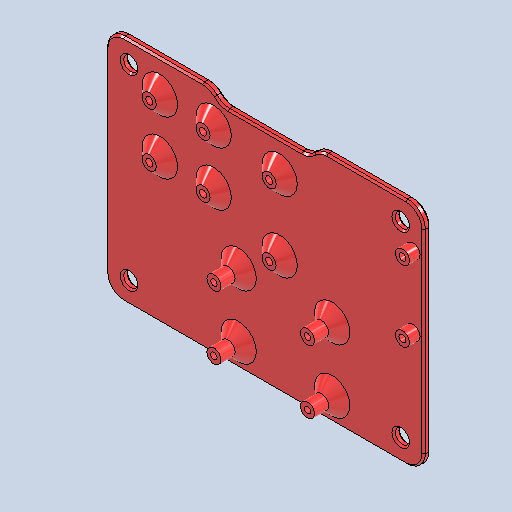
# Autodesk Inventor part: temp-logger-shelf-v2
Saved by Autodesk Inventor 2026 (Build 300175050, 175E)
## iProperties
Created: 2025-07-16
Part Number: temp-logger-shelf-v2
Material: ABS Plastic
Document SubType Name: Modeling
Designer: kuzmin
Density: 1.06 g/cm^3
Appearance: Light Red
Author: kuzmin
Autodesk Inventor part; units mm, degrees
ref_plane "YZ Plane" through (0, 0, 0) normal (1, 0, 0) x (0, 1, 0)
ref_plane "XZ Plane" through (0, 0, 0) normal (0, 1, 0) x (-1, 0, 0)
ref_plane "XY Plane" through (0, 0, 0) normal (0, 0, 1) x (1, 0, 0)
sketch "Sketch1" plane through (0, 0, 0) normal (0, 0, 1) x (1, 0, 0)
  line L0 (-45, 32.5) -> (45, 32.5)
  line L1 (45, 32.5) -> (45, -32.5)
  line L2 (45, -32.5) -> (-45, -32.5)
  line L3 (-45, -32.5) -> (-45, 32.5)
  line L4 (-38.5, 26.5) -> (38.5, 26.5) construction
  line L5 (38.5, 26.5) -> (38.5, -26.5) construction
  line L6 (38.5, -26.5) -> (-38.5, -26.5) construction
  line L7 (-38.5, -26.5) -> (-38.5, 26.5) construction
  circle A0 centre (-38.5, 26.5) radius 2
  circle A1 centre (38.5, 26.5) radius 2
  circle A2 centre (38.5, -26.5) radius 2
  circle A3 centre (-38.5, -26.5) radius 2
  point P0 (0, 0)
  point P1 (45, 0)
  point P2 (0, 32.5)
  point P3 (38.5, 0)
  point P4 (0, 26.5)
  dimension "d0" = 90
  dimension "d1" = 65
  dimension "d2" = 77
  dimension "d3" = 53
  dimension "d14" = 4
  constraints: 16 end point, 8 coincident, 4 centre point, 4 midpoint, 4 parallel, 3 equal radius, 2 horizontal, 2 horizontal alignment, 2 perpendicular, 2 vertical alignment
  measures "d0" distance of L0.start L0.end
  measures "d1" distance of L0.end L1.end
  measures "d2" distance of L4.start L4.end
  measures "d3" distance of L4.end L5.end
  measures "d14" diameter of A0
extrude "Extrusion1" add sketch "Sketch1" along normal blind 2 contours L0 L1 L2 L3 | A0 | A1 | A2 | A3
hole "Hole1" at (38.5, 26.5, 0) at (38.5, -26.5, 0) at (-38.5, -26.5, 0) at (-38.5, 26.5, 0) direction (0, 0, 1) diameter 4 end through all
sketch "Sketch3" plane through (0, 0, 0) normal (0, 0, -1) x (-1, 0, 0)
  line L0 (-42, 21) -> (-4.2, 21) construction
  line L1 (-4.2, 21) -> (-4.2, 1) construction
  line L2 (-4.2, 1) -> (-42, 1) construction
  line L3 (-42, 1) -> (-42, 21) construction
  circle A0 centre (-42, 21) radius 2
  circle A1 centre (-4.2, 21) radius 2
  circle A2 centre (-4.2, 1) radius 2
  circle A3 centre (-42, 1) radius 2
  line L4 (-40, -32.5) -> (40, -32.5) projected
  line L5 (-45, -32.5) -> (-45, 32.5) projected
  point P0 (0, 0)
  point P1 (-4.2, 11)
  point P2 (-45, -27.5)
  point P3 (-45, 27.5)
  dimension "d27" = 20
  dimension "d28" = 37.8
  dimension "d30" = 4
  dimension "d47" = 3
  dimension "d107" = 21
  constraints: 8 coincident, 8 end point, 4 centre point, 3 equal radius, 2 parallel, 1 horizontal, 1 midpoint, 1 perpendicular
  measures "d27" distance of L0.end L1.end
  measures "d28" distance of L0.start L0.end
  measures "d30" diameter of A1
  measures "d47" distance between parallel lines of L5 L3
  measures "d107" distance from line of point (0, 0) L0
extrude "Extrusion4" add sketch "Sketch3" against normal blind 5
hole "Hole2" at (4.2, 21, 0) at (4.2, 1, 0) at (42, 1, 0) at (42, 21, 0) direction (0, 0, 1) diameter 2 end through all
sketch "Sketch8" plane through (0, 0, 2) normal (0, 0, 1) x (1, 0, 0)
  line L0 (45, 32.5) -> (-45, 32.5) projected
  line L1 (-15, 32.5) -> (15, 32.5)
  line L2 (15, 32.5) -> (15, 29.5)
  line L3 (15, 29.5) -> (-15, 29.5)
  line L4 (-15, 29.5) -> (-15, 32.5)
  point P0 (0, 0)
  point P1 (0, 29.5)
  dimension "d108" = 30
  dimension "d109" = 3
  constraints: 8 end point, 2 parallel, 1 horizontal, 1 midpoint, 1 perpendicular, 1 point on line, 1 vertical alignment
  measures "d108" distance of L2.end L3.end
  measures "d109" distance of L3.end L1.start
extrude "Extrusion10" cut sketch "Sketch8" against normal through all
chamfer "Chamfer3" distance 3 angle 45 2 edges at (6.2, 21, 2) (6.2, 1, 2)
fillet "Fillet2" radius 5 8 edges at (-45, 32.5, 1) (-45, -32.5, 1) (45, -32.5, 1) (45, 32.5, 1) (-15, 32.5, 1) (-15, 29.5, 1) (15, 29.5, 1) (15, 32.5, 1)
chamfer "Chamfer5" distance 0.5 angle 45 34 edges at (0, -32.5, 2) (43.5355, -31.0355, 2) (-43.5355, -31.0355, 2) (12.3539, 29.8902, 2) (15.6224, 32.1098, 2) (43.5355, 31.0355, 2) (-43.5355, 31.0355, 2) (-15.6224, 32.1098, 2) (-12.3539, 29.8902, 2) (45, 0, 2) (28.7794, 32.5, 2) (-28.7794, 32.5, 2) (-45, 0, 2) (43.5355, 31.0355, 0) (28.7794, 32.5, 0) (-28.7794, 32.5, 0) (-43.5355, 31.0355, 0) (-45, 0, 0) (-43.5355, -31.0355, 0) (0, -32.5, 0) (43.5355, -31.0355, 0) (12.3539, 29.8902, 0) (15.6224, 32.1098, 0) (-15.6224, 32.1098, 0) (-12.3539, 29.8902, 0) (45, 0, 0) (-38.5, 24.5, 2) (-38.5, -28.5, 2) (38.5, -28.5, 2) (38.5, 24.5, 2) (-38.5, 24.5, 0) (38.5, 24.5, 0) (38.5, -28.5, 0) (-38.5, -28.5, 0)
sketch "Sketch6" plane through (0, 0, 2) normal (0, 0, 1) x (1, 0, 0)
  line L0 (-7.4152, -8) -> (19.0848, -8) construction
  line L1 (19.0848, -8) -> (19.0848, -26) construction
  line L2 (19.0848, -26) -> (-7.4152, -26) construction
  line L3 (-7.4152, -26) -> (-7.4152, -8) construction
  line L4 (-20, 12.5) -> (-20, -12.5) projected
  circle A0 centre (-7.4152, -8) radius 2
  circle A1 centre (-7.4152, -26) radius 2
  circle A2 centre (19.0848, -26) radius 2
  circle A3 centre (-7.4152, -8) radius 0.9
  circle A4 centre (-7.4152, -26) radius 0.9
  circle A5 centre (19.0848, -26) radius 0.9
  circle A6 centre (19.0848, -8) radius 0.9
  circle A7 centre (19.0848, -8) radius 2
  point P0 (0, 0)
  dimension "d73" = 18
  dimension "d74" = 26.5
  dimension "d77" = 4
  dimension "d80" = 1.8
  dimension "d90" = 8
  constraints: 11 coincident, 8 centre point, 8 end point, 6 equal radius, 2 parallel, 1 horizontal, 1 perpendicular
  measures "d73" distance of L2.end L0.start
  measures "d74" distance of L0.start L0.end
  measures "d77" diameter of A2
  measures "d80" diameter of A3
  measures "d90" distance from line of point (0, 0) L0
extrude "Extrusion6" add sketch "Sketch6" along normal blind 7
chamfer "Chamfer9" distance 3 angle 45 4 edges at (17.0848, -8, 2) (17.0848, -26, 2) (-9.4152, -8, 2) (-9.4152, -26, 2)
sketch "Sketch7" plane through (0, 0, 2) normal (0, 0, 1) x (1, 0, 0)
  line L0 (-14.497, 23.5115) -> (-29.737, 23.5115) construction
  line L1 (-29.737, 23.5115) -> (-29.737, 8.2715) construction
  line L2 (-29.737, 8.2715) -> (-14.497, 8.2715) construction
  line L3 (-14.497, 8.2715) -> (-14.497, 23.5115) construction
  circle A0 centre (-14.497, 23.5115) radius 1
  circle A1 centre (-14.497, 8.2715) radius 1
  circle A2 centre (-29.737, 8.2715) radius 1
  circle A3 centre (-29.737, 23.5115) radius 1
  circle A4 centre (-14.497, 23.5115) radius 2
  circle A5 centre (-29.737, 23.5115) radius 2
  circle A6 centre (-14.497, 8.2715) radius 2
  circle A7 centre (-29.737, 8.2715) radius 2
  point P0 (0, 0)
  dimension "d96" = 15.24
  dimension "d98" = 2
  dimension "d99" = 4
  constraints: 8 centre point, 8 coincident, 8 end point, 6 equal radius, 2 parallel, 2 perpendicular, 1 horizontal
  measures "d96" distance of L1.end L2.end
  measures "d98" diameter of A0
  measures "d99" diameter of A4
extrude "Extrusion8" add sketch "Sketch7" along normal blind 3
chamfer "Chamfer10" distance 3 angle 45 4 edges at (-16.497, 23.5115, 2) (-16.497, 8.2715, 2) (-31.737, 8.2715, 2) (-31.737, 23.5115, 2)
extrude "Extrusion9" cut sketch "Sketch7" against normal through all contours A0 | A1 | A2 | A3
equation "\"d4\" = thickness"
equation "\"d31\" = thickness + bump"
equation "\"thickness\" = 2"
equation "\"bump\" = 3"
body "Solid1"
